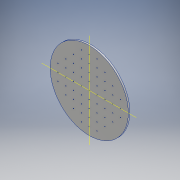
# Autodesk Inventor part: circularBaseplate
Saved by Autodesk Inventor 2017 SP1 (Build 210196100, 196)
## iProperties
Created: 2018-05-03
Part Number: circularBaseplate
Material: Aluminum 6061
Document SubType Name: Modeling
Designer: Sam
Density: 2.7 g/cm^3
Appearance: Aluminum - Flat
Mass: 5272.21 g
Surface Area: 4150.47 cm^2
Volume: 1952.67 cm^3
Author: Sam
Autodesk Inventor part; units mm, degrees
sketch "Sketch1" plane through (0, 0, 0) normal (0, 1, 0) x (-1, 0, 0)
  circle A0 centre (0, 0) radius 250
  dimension "d0" = 500
  constraints: 1 centre point, 1 coincident
  measures "d0" diameter of A0
extrude "Extrusion1" add sketch "Sketch1" along normal blind 10
sketch "Sketch2" plane through (0, 10, 0) normal (0, 1, 0) x (1, 0, 0)
  point P0 (0, 0)
  point P1 (-50, -200)
  point P2 (0, -200)
  point P3 (50, -200)
  point P4 (-100, -150)
  point P5 (-50, -150)
  point P6 (0, -150)
  point P7 (50, -150)
  point P8 (100, -150)
  point P9 (-150, -100)
  point P10 (-100, -100)
  point P11 (-50, -100)
  point P12 (0, -100)
  point P13 (50, -100)
  point P14 (100, -100)
  point P15 (150, -100)
  point P16 (-200, -50)
  point P17 (-150, -50)
  point P18 (-100, -50)
  point P19 (-50, -50)
  point P20 (0, -50)
  point P21 (50, -50)
  point P22 (100, -50)
  point P23 (150, -50)
  point P24 (200, -50)
  point P25 (-200, 0)
  point P26 (-150, 0)
  point P27 (-100, 0)
  point P28 (-50, 0)
  point P29 (0, 0)
  point P30 (50, 0)
  point P31 (100, 0)
  point P32 (150, 0)
  point P33 (200, 0)
  point P34 (-200, 50)
  point P35 (-150, 50)
  point P36 (-100, 50)
  point P37 (-50, 50)
  point P38 (0, 50)
  point P39 (50, 50)
  point P40 (100, 50)
  point P41 (150, 50)
  point P42 (200, 50)
  point P43 (-150, 100)
  point P44 (-100, 100)
  point P45 (-50, 100)
  point P46 (0, 100)
  point P47 (50, 100)
  point P48 (100, 100)
  point P49 (150, 100)
  point P50 (-100, 150)
  point P51 (-50, 150)
  point P52 (0, 150)
  point P53 (50, 150)
  point P54 (100, 150)
  point P55 (-50, 200)
  point P56 (0, 200)
  point P57 (50, 200)
hole "Hole1" at (-50, 10, 200) at (0, 10, 200) at (50, 10, 200) at (-100, 10, 150) at (-50, 10, 150) at (0, 10, 150) at (50, 10, 150) at (100, 10, 150) at (-150, 10, 100) at (-100, 10, 100) at (-50, 10, 100) at (0, 10, 100) at (50, 10, 100) at (100, 10, 100) at (150, 10, 100) at (-200, 10, 50) at (-150, 10, 50) at (-100, 10, 50) at (-50, 10, 50) at (0, 10, 50) at (50, 10, 50) at (100, 10, 50) at (150, 10, 50) at (200, 10, 50) at (-200, 10, 0) at (-150, 10, 0) at (-100, 10, 0) at (-50, 10, 0) at (0, 10, 0) at (50, 10, 0) at (100, 10, 0) at (150, 10, 0) at (200, 10, 0) at (-200, 10, -50) at (-150, 10, -50) at (-100, 10, -50) at (-50, 10, -50) at (0, 10, -50) at (50, 10, -50) at (100, 10, -50) at (150, 10, -50) at (200, 10, -50) at (-150, 10, -100) at (-100, 10, -100) at (-50, 10, -100) at (0, 10, -100) at (50, 10, -100) at (100, 10, -100) at (150, 10, -100) at (-100, 10, -150) direction (0, -1, 0) diameter 4.917 end through all and at (-50, 10, -150) (0, 10, -150) (50, 10, -150) (100, 10, -150) (-50, 10, -200) (0, 10, -200) (50, 10, -200) thread size "M6x1" class "6H" standard "ISO Metric profile"
body "Solid1"
